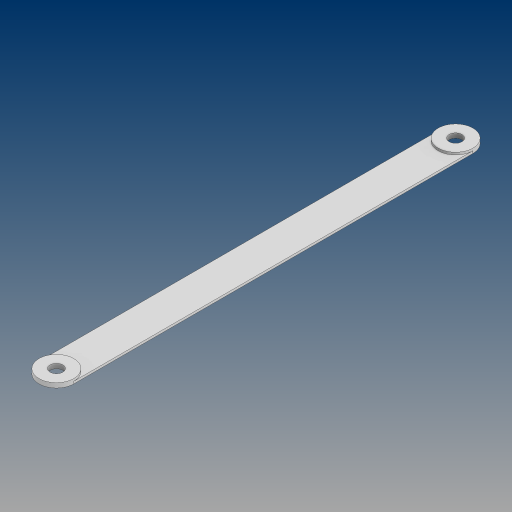
# Autodesk Inventor part: kozepsoszalag2
Saved by Autodesk Inventor 2023 (Build 270158000, 158)
## iProperties
Created: 2023-11-15
Part Number: kozepsoszalag2
Material: Generic
Document SubType Name: Modeling
Designer: gd1
Density: 1 g/cm^3
Appearance: Default
Author: gd1
Autodesk Inventor part; units mm, degrees
ref_plane "YZ Plane" through (0, 0, 0) normal (1, 0, 0) x (0, 1, 0)
ref_plane "XZ Plane" through (0, 0, 0) normal (0, 1, 0) x (-1, 0, 0)
ref_plane "XY Plane" through (0, 0, 0) normal (0, 0, 1) x (1, 0, 0)
sketch "Sketch1" plane through (0, 0, 0) normal (0, 1, 0) x (-1, 0, 0)
  line L0 (0, 0) -> (0, -157.6812)
  line L1 (0, 0) -> (157.6812, 0) construction
  line L2 (0, 0) -> (7.5, 0)
  line L3 (7.5, 0) -> (-7.5, 0)
  line L4 (-7.5, 0) -> (-7.5, -15)
  line L5 (-7.5, -15) -> (7.5, -15)
  line L6 (7.5, -15) -> (7.5, 0)
  circle A0 centre (0, -7.5) radius 7.5
  line L7 (-7.5, -78.8406) -> (7.5, -78.8406)
  circle A1 centre (0, -150.1812) radius 7.5
  line L8 (-7.5, 0) -> (7.5, 0)
  line L9 (7.5, 0) -> (7.5, -157.6812)
  line L10 (7.5, -157.6812) -> (-7.5, -157.6812)
  line L11 (-7.5, -157.6812) -> (-7.5, 0)
  circle A2 centre (0, -7.5) radius 2.75
  circle A3 centre (0, -150.1812) radius 2.75
  line L12 (7.5, 0) -> (-7.5, 0)
  line L13 (-7.5, 0) -> (-7.5, 15)
  line L14 (-7.5, 15) -> (7.5, 15)
  line L15 (7.5, 15) -> (7.5, 0)
  line L16 (7.5, -157.6812) -> (-7.5, -157.6812)
  line L17 (-7.5, -157.6812) -> (-7.5, -172.6812)
  line L18 (-7.5, -172.6812) -> (7.5, -172.6812)
  line L19 (7.5, -172.6812) -> (7.5, -157.6812)
  circle A4 centre (0, 7.5) radius 7.5
  circle A5 centre (0, -165.1812) radius 7.5
  circle A6 centre (0, 7.5) radius 2.75
  circle A7 centre (0, -165.1812) radius 2.75
  point P0 (7.5, -7.5)
  point P1 (-7.5, -7.5)
  point P2 (-7.5, -150.1812)
  point P3 (7.5, -150.1812)
  point P4 (-7.5, -165.1812)
  point P5 (7.5, -165.1812)
  point P6 (7.5, 7.5)
  point P7 (-7.5, 7.5)
  dimension "d0" = 157.6812
  dimension "d1" = 90
  dimension "d2" = 7.5
  dimension "d3" = 15
  dimension "d4" = 15
  dimension "d5" = 5.5
  dimension "d6" = 5.5
  dimension "d11" = 15
  dimension "d12" = 15
  dimension "d13" = 5.5
  dimension "d14" = 5.5
  constraints: 40 end point, 8 centre point, 8 parallel, 6 horizontal, 5 perpendicular, 4 coincident, 2 point on line, 1 symmetric about line, 1 tangent, 1 vertical, 1 other
  measures "d0" distance of L0.start L0.end
  measures "d1" angle of L0 L1
  measures "d2" distance of L0.start L2.end
  measures "d3" distance of L5.end L4.end
  measures "d4" distance of L4.end L3.end
  measures "d5" diameter of A2
  measures "d6" diameter of A3
  measures "d11" distance of L12.end L13.end
  measures "d12" distance of L17.end L16.end
  measures "d13" diameter of A6
  measures "d14" diameter of A7
extrude "Extrusion1" add sketch "Sketch1" along normal blind 1 contours A0 L0 A2 | A4 L15 L2 | A0 L4 L3 | L2 L6 A0 | L0 A2 A0 | A4 | L3 L13 A4 | A2 L0 | L0 A2 | L6 L5 A0 | A0 L5 L4 | L9 L7 L0 L5 | L0 L7 L11 L5 | L9 A1 L0 L7 | L0 A1 L11 L7 | L9 L10 A1 | A1 L0 A3 | L0 A3 A1 | A1 L10 L11 | A5 L17 L10 | L10 L19 A5 | A5 | A3 L0 | L0 A3
extrude "Extrusion2" add sketch "Sketch1" along normal blind 2 contours A4 | A5
body "Solid1"
